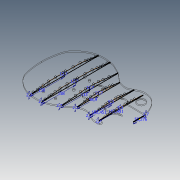
# Autodesk Inventor part: Tampo2
Saved by Autodesk Inventor 2016 (Build 200138000, 138)
## iProperties
Created: 2018-10-29
Part Number: Tampo2
Material: Generic
Document SubType Name: Modeling
Designer: Pedro Mendonça
Density: 1 g/cm^3
Appearance: Default
Author: Pedro Mendonça
Autodesk Inventor part; units mm, degrees
ref_plane "YZ Plane" through (0, 0, 0) normal (1, 0, 0) x (0, 1, 0)
ref_plane "XY Plane" through (0, 0, 0) normal (0, 0, 1) x (1, 0, 0)
sketch "Sketch1" plane through (0, 0, 0) normal (0, 0, 1) x (1, 0, 0)
  circle A0 centre (34.423, -78.21) radius 1
  circle A1 centre (41.5, -294) radius 4.5
  circle A2 centre (-41.5, -294) radius 4.5
  circle A3 centre (-36.7, -267.7941) radius 4.5
  circle A4 centre (36.7, -267.7941) radius 4.5
  line L0 (35, -127.21) -> (-13.5738, -127.21)
  line L1 (33.9001, -190.21) -> (35, -190.21)
  arc A5 (39, -194.21) -> (35, -190.21) centre (35, -194.21) ccw
  line L2 (39, -194.21) -> (39, -196.9778)
  line L3 (41.0589, -199.71) -> (41.5, -199.71)
  arc A6 (43.5, -201.71) -> (41.5, -199.71) centre (41.5, -201.71) ccw
  line L4 (43.5, -201.71) -> (43.5, -202.9495)
  arc A7 (35, -232.21) -> (38.6777, -229.783) centre (35, -228.21) ccw
  line L5 (35, -232.21) -> (-35, -232.21)
  arc A8 (-39, -228.21) -> (-35, -232.21) centre (-35, -228.21) ccw
  line L6 (-39, -228.21) -> (-39, -224.71)
  arc A9 (-39, -224.71) -> (-41, -222.71) centre (-41, -224.71) ccw
  line L7 (-41, -222.71) -> (-41.5, -222.71)
  arc A10 (-43.5, -220.71) -> (-41.5, -222.71) centre (-41.5, -220.71) ccw
  line L8 (-43.5, -220.71) -> (-43.5, -201.71)
  arc A11 (-41.5, -199.71) -> (-43.5, -201.71) centre (-41.5, -201.71) ccw
  line L9 (-41.5, -199.71) -> (-41, -199.71)
  arc A12 (-41, -199.71) -> (-39, -197.71) centre (-41, -197.71) ccw
  line L10 (-39, -197.71) -> (-39, -194.21)
  arc A13 (-35, -190.21) -> (-39, -194.21) centre (-35, -194.21) ccw
  line L11 (-35, -190.21) -> (8.8574, -190.21)
  arc A14 (-55.8091, -71.1619) -> (-75.5317, -78.2219) centre (-70.5, -61.2) ccw
  arc A15 (-39.1003, -93.3353) -> (-39, -92.71) centre (-41, -92.71) ccw
  line L12 (-39, -92.71) -> (-39, -89.21)
  arc A16 (-35, -85.21) -> (-39, -89.21) centre (-35, -89.21) ccw
  line L13 (-35, -85.21) -> (-28.53, -85.21)
  line L14 (-28.53, -85.21) -> (-27.2617, -2.2163)
  spline S0 degree 4 poles (-27.2617, -2.2163) (-43.8413, -5.0737) (-69.2989, -15.2577) (-85.7631, -26.5127) (-99.6977, -40.3072) (-106.7365, -51.5397) (-111.6352, -63.1761) (-114.1418, -74.0378) (-115.9364, -86.2479) (-114.7925, -100.8201) (-111.1925, -111.3398) (-104.9533, -123.6353) (-99.2411, -132.3298) (-94.3304, -141.7669) (-90.7434, -152.656) (-92.8358, -167.4735) (-95.3552, -177.4658) (-100.5222, -191.8137) (-106.2015, -200.3968) (-115.9364, -209.2361) (-126.4423, -222.6445) (-135, -233.5666) (-138.9752, -242.9989) (-144.1012, -253.4714) (-148.4765, -261.546) (-152.3095, -270.0787) (-155.7121, -278.8181) (-157.4845, -291.3466) (-158.9541, -299.1238) (-160.7041, -310.0555) (-161.3959, -321.0408) (-160.2622, -336.1037) (-159.5472, -351.6393) (-155.7121, -363.9428) (-152.044, -373.8933) (-146.9896, -384.4071) (-140.8913, -395.5086) (-132.7759, -406.8471) (-124.2149, -416.631) (-110.5874, -430.5207) (-101.5897, -436.4609) (-90.9559, -441.7244) (-72.5, -447.3805) (-55.0288, -449.8264) (-39.9161, -452.9713) (-21.0472, -455.5046) (0, -455) knots 1.260865 1.260865 1.260865 1.260865 1.260865 2 2.830975 3 3.639707 4 5 5.266438 6 6.852799 7 7.750355 8 8.949877 9 10 10.263862 11 11.607775 12 12.940348 13 13.693379 14 14.438323 15 15.641425 16 16.183585 17 18 19 19.17802 19.513385 20 20.856717 21 21.323358 21.522075 21.533515 21.674547 21.764236 21.807897 22 22 22 22 22
  spline S1 degree 4 poles (0, -455) (21.0472, -455.5046) (39.9161, -452.9713) (55.0288, -449.8264) (72.5, -447.3805) (90.9559, -441.7244) (101.5897, -436.4609) (110.5874, -430.5207) (124.2149, -416.631) (132.7759, -406.8471) (140.8913, -395.5086) (146.9896, -384.4071) (152.044, -373.8933) (155.7121, -363.9428) (159.5472, -351.6393) (160.2622, -336.1037) (161.3959, -321.0408) (160.7041, -310.0555) (158.9541, -299.1238) (157.4845, -291.3466) (155.7121, -278.8181) (152.3095, -270.0787) (148.4765, -261.546) (144.1012, -253.4714) (138.9752, -242.9989) (135, -233.5666) (126.4423, -222.6445) (115.9364, -209.2361) (106.2015, -200.3968) (100.5222, -191.8137) (95.3552, -177.4658) (92.8358, -167.4735) (90.7434, -152.656) (94.3304, -141.7669) (99.2411, -132.3298) (104.9533, -123.6353) (111.1925, -111.3398) (114.7925, -100.8201) (115.7876, -88.1434) (114.9001, -79.7366) (114.1554, -75.2406) (113.4907, -72.1039) knots 1 1 1 1 1 1.192103 1.235764 1.325453 1.466485 1.477925 1.676642 2 2.143283 3 3.486615 3.82198 4 5 6 6.816415 7 7.358575 8 8.561677 9 9.306621 10 10.059652 11 11.392225 12 12.736138 13 14 14.050123 15 15.249645 16 16.147201 17 17.733562 18 18.628908 18.628908 18.628908 18.628908 18.628908
  arc A17 (113.4907, -72.1039) -> (102.4514, -70.3024) centre (107.621, -73.3478) ccw
  arc A18 (28.0139, -51.4408) -> (102.4514, -70.3024) centre (67.9874, -50) ccw
  line L15 (28.0139, -51.4408) -> (28.53, -85.21)
  line L16 (28.53, -85.21) -> (35, -85.21)
  arc A19 (39, -89.21) -> (35, -85.21) centre (35, -89.21) ccw
  line L17 (39, -89.21) -> (39, -92.71)
  arc A20 (39, -92.71) -> (41, -94.71) centre (41, -92.71) ccw
  line L18 (41, -94.71) -> (41.5, -94.71)
  arc A21 (43.5, -96.71) -> (41.5, -94.71) centre (41.5, -96.71) ccw
  line L19 (43.5, -96.71) -> (43.5, -115.71)
  arc A22 (41.5, -117.71) -> (43.5, -115.71) centre (41.5, -115.71) ccw
  line L20 (41.5, -117.71) -> (41, -117.71)
  arc A23 (41, -117.71) -> (39, -119.71) centre (41, -119.71) ccw
  line L21 (39, -119.71) -> (39, -123.21)
  arc A24 (35, -127.21) -> (39, -123.21) centre (35, -123.21) ccw
  line L22 (-39, -123.21) -> (-39, -119.71)
  arc A25 (-39, -123.21) -> (-35, -127.21) centre (-35, -123.21) ccw
  line L23 (35, -127.21) -> (-35, -127.21)
  arc A26 (35, -127.21) -> (39, -123.21) centre (35, -123.21) ccw
  line L24 (39, -119.71) -> (39, -123.21)
  arc A27 (41, -117.71) -> (39, -119.71) centre (41, -119.71) ccw
  line L25 (41.5, -117.71) -> (41, -117.71)
  arc A28 (41.5, -117.71) -> (43.5, -115.71) centre (41.5, -115.71) ccw
  line L26 (43.5, -96.71) -> (43.5, -115.71)
  arc A29 (43.5, -96.71) -> (41.5, -94.71) centre (41.5, -96.71) ccw
  line L27 (41, -94.71) -> (41.5, -94.71)
  arc A30 (39, -92.71) -> (41, -94.71) centre (41, -92.71) ccw
  line L28 (39, -89.21) -> (39, -92.71)
  arc A31 (39, -89.21) -> (35, -85.21) centre (35, -89.21) ccw
  arc A32 (-35, -85.21) -> (-39, -89.21) centre (-35, -89.21) ccw
  line L29 (-39, -92.71) -> (-39, -89.21)
  arc A33 (-41, -94.71) -> (-39, -92.71) centre (-41, -92.71) ccw
  line L30 (-41.5, -94.71) -> (-41, -94.71)
  arc A34 (-41.5, -94.71) -> (-43.5, -96.71) centre (-41.5, -96.71) ccw
  line L31 (-43.5, -115.71) -> (-43.5, -96.71)
  arc A35 (-43.5, -115.71) -> (-41.5, -117.71) centre (-41.5, -115.71) ccw
  line L32 (-41, -117.71) -> (-41.5, -117.71)
  arc A36 (-39, -119.71) -> (-41, -117.71) centre (-41, -119.71) ccw
  line L33 (-39, -228.21) -> (-39, -224.71)
  arc A37 (-39, -228.21) -> (-35, -232.21) centre (-35, -228.21) ccw
  line L34 (35, -232.21) -> (-35, -232.21)
  arc A38 (35, -232.21) -> (39, -228.21) centre (35, -228.21) ccw
  line L35 (39, -224.71) -> (39, -228.21)
  arc A39 (41, -222.71) -> (39, -224.71) centre (41, -224.71) ccw
  line L36 (41.5, -222.71) -> (41, -222.71)
  arc A40 (41.5, -222.71) -> (43.5, -220.71) centre (41.5, -220.71) ccw
  line L37 (43.5, -201.71) -> (43.5, -220.71)
  arc A41 (43.5, -201.71) -> (41.5, -199.71) centre (41.5, -201.71) ccw
  line L38 (41, -199.71) -> (41.5, -199.71)
  arc A42 (39, -197.71) -> (41, -199.71) centre (41, -197.71) ccw
  line L39 (39, -194.21) -> (39, -197.71)
  arc A43 (39, -194.21) -> (35, -190.21) centre (35, -194.21) ccw
  line L40 (-35, -190.21) -> (35, -190.21)
  arc A44 (-35, -190.21) -> (-39, -194.21) centre (-35, -194.21) ccw
  line L41 (-39, -197.71) -> (-39, -194.21)
  arc A45 (-41, -199.71) -> (-39, -197.71) centre (-41, -197.71) ccw
  line L42 (-41.5, -199.71) -> (-41, -199.71)
  arc A46 (-41.5, -199.71) -> (-43.5, -201.71) centre (-41.5, -201.71) ccw
  line L43 (-43.5, -220.71) -> (-43.5, -201.71)
  arc A47 (-43.5, -220.71) -> (-41.5, -222.71) centre (-41.5, -220.71) ccw
  line L44 (-41, -222.71) -> (-41.5, -222.71)
  arc A48 (-39, -224.71) -> (-41, -222.71) centre (-41, -224.71) ccw
  arc A49 (-55.8091, -71.1619) -> (-75.5317, -78.2219) centre (-70.5, -61.2) ccw
  arc A50 (-75.5317, -78.2219) -> (-55.8091, -71.1619) centre (-70.5, -61.2) ccw
  circle A51 centre (74, -297.4128) radius 3.7
  circle A52 centre (113.9223, -275.0602) radius 3.7
  circle A53 centre (113.9223, -331.1092) radius 3.7
  circle A54 centre (74, -348.8838) radius 3.7
  line L45 (-35, -85.21) -> (-28.53, -85.21)
  line L46 (28.53, -85.21) -> (35, -85.21)
  point P0 (0, 0)
  point P1 (0, 0)
  constraints: 94 end point, 92 point on circle, 55 centre point, 4 other
extrude "base" add sketch "Sketch1" along normal blind 5.4
ref_plane "Work Plane1" through (-28.53, -85.21, 5.4) normal (0, 1, 0) x (-1, 0, 0)
ref_plane "Work Plane2" through (0, -127.21, 5.4) normal (0, 1, 0) x (-1, 0, 0)
ref_plane "Work Plane3" through (0, -190.21, 0) normal (0, 1, 0) x (-1, 0, 0)
ref_plane "Work Plane4" through (0, -232.21, 0) normal (0, 1, 0) x (-1, 0, 0)
ref_plane "Work Plane5" through (41.5, -294, 5.4) normal (0, 1, 0) x (-1, 0, 0)
ref_plane "Work Plane6" through (74, -348.8838, 0) normal (0, 1, 0) x (-1, 0, 0)
sketch "Sketch2" plane through (0, 0, 0) normal (0, 1, 0) x (-1, 0, 0)
  line L0 (-28.0139, 5.4) -> (27.2617, 5.4)
  line L1 (27.2617, 5.4) -> (27.2617, 2.7)
  line L2 (-28.0139, 5.4) -> (-28.0139, 2.7)
  line L3 (-28.0139, 2.7) -> (27.2617, 2.7)
  point P0 (0, 0)
  dimension "d45" = 2.7
  dimension "d46" = 55.2756
  constraints: 8 end point, 2 horizontal, 1 perpendicular, 1 point on line
  measures "d45" distance of L0.end L1.end
  measures "d46" distance of L2.end L1.end
sketch "Sketch3" plane through (-28.53, -85.21, 5.4) normal (0, 1, 0) x (-1, 0, 0)
  line L0 (-28.53, -2.7) -> (-28.53, 2.6)
  line L1 (-28.53, -2.7) -> (-28.53, 0)
  line L2 (-28.53, 0) -> (-131.03, 0) construction
  line L3 (-130.9814, -2.7) -> (-130.9814, 0)
  line L4 (-130.9814, 0) -> (-90.7981, 1.127) construction
  line L5 (-90.7981, 1.127) -> (-77.2588, 1.5284) construction
  line L6 (-77.2588, 1.5284) -> (-60.9572, 1.5284) construction
  line L7 (-60.9572, 1.5284) -> (-46.9035, 2.6) construction
  line L8 (-46.9035, 2.6) -> (-28.53, 2.6) construction
  spline S0 degree 4 poles (-130.9814, 0) (-90.7981, 1.127) (-77.2588, 1.5284) (-60.9572, 1.5284) (-46.9035, 2.6) (-28.53, 2.6) knots 1 1 1 1 1 2 3 3 3 3 3
  line L9 (-130.9814, 0) -> (-130.9814, -2.7)
  line L10 (-130.9814, 0) -> (-125.5814, 0) construction
  line L11 (-130.9814, -2.7) -> (-28.53, -2.7)
  line L12 (-28.53, 0) -> (73.97, 0) construction
  line L13 (73.9214, -2.7) -> (73.9214, 0)
  line L14 (73.9214, 0) -> (33.7381, 1.127) construction
  spline S1 degree 4 poles (73.9214, 0) (33.7381, 1.127) (20.1988, 1.5284) (3.8972, 1.5284) (-10.1565, 2.6) (-28.53, 2.6) knots 1 1 1 1 1 2 3 3 3 3 3
  line L15 (33.7381, 1.127) -> (20.1988, 1.5284) construction
  line L16 (20.1988, 1.5284) -> (3.8972, 1.5284) construction
  line L17 (3.8972, 1.5284) -> (-10.1565, 2.6) construction
  line L18 (-10.1565, 2.6) -> (-28.53, 2.6) construction
  line L19 (73.9214, 0) -> (73.9214, -2.7)
  line L20 (73.9214, 0) -> (68.5214, 0) construction
  line L21 (73.9214, -2.7) -> (-28.53, -2.7)
  point P0 (-28.53, -5.4)
  dimension "d42" = 5.3
  dimension "d43" = 102.4514
  dimension "d44" = 2.7
  constraints: 24 end point, 8 symmetric about line, 3 horizontal, 1 collinear, 1 vertical, 6 other
  measures "d42" distance of L0.start L0.end
  measures "d43" distance of L3.start L0.start
  measures "d44" distance of L3.end L3.start
sketch "Sketch5" plane through (0, -127.21, 5.4) normal (0, 1, 0) x (-1, 0, 0)
  line L0 (0, -2.7) -> (0, 6.6)
  line L1 (0, 0) -> (-102.5, 0) construction
  line L2 (-102.4514, 0) -> (-60.1171, 1.5284) construction
  line L3 (-60.1171, 1.5284) -> (-42.8591, 3.5935) construction
  line L4 (-42.8591, 3.5935) -> (-28.8463, 5.806) construction
  line L5 (-28.8463, 5.806) -> (-18.3735, 6.6) construction
  line L6 (-18.3735, 6.6) -> (0, 6.6) construction
  spline S0 degree 4 poles (-102.4514, 0) (-60.1171, 1.5284) (-42.8591, 3.5935) (-28.8463, 5.806) (-18.3735, 6.6) (0, 6.6) knots 1 1 1 1 1 2 3 3 3 3 3
  line L7 (-102.4514, 0) -> (-102.4514, -2.7)
  line L8 (-102.4514, 0) -> (-97.0514, 0) construction
  line L9 (-102.4514, -2.7) -> (0, -2.7)
  line L10 (0, 0) -> (102.5, 0) construction
  line L11 (102.4514, 0) -> (60.1171, 1.5284) construction
  line L12 (60.1171, 1.5284) -> (42.8591, 3.5935) construction
  line L13 (42.8591, 3.5935) -> (28.8463, 5.806) construction
  line L14 (28.8463, 5.806) -> (18.3735, 6.6) construction
  line L15 (18.3735, 6.6) -> (0, 6.6) construction
  spline S1 degree 4 poles (102.4514, 0) (60.1171, 1.5284) (42.8591, 3.5935) (28.8463, 5.806) (18.3735, 6.6) (0, 6.6) knots 1 1 1 1 1 2 3 3 3 3 3
  line L16 (102.4514, 0) -> (102.4514, -2.7)
  line L17 (102.4514, 0) -> (97.0514, 0) construction
  line L18 (102.4514, -2.7) -> (0, -2.7)
  dimension "d39" = 102.4514
  dimension "d40" = 9.3
  dimension "d41" = 2.7
  constraints: 18 end point, 8 symmetric about line, 3 horizontal, 1 vertical, 6 other
  measures "d39" distance of L7.end L0.start
  measures "d40" distance of L0.start L0.end
  measures "d41" distance of L2.start L7.end
sketch "Sketch6" plane through (0, -190.21, 0) normal (0, 1, 0) x (-1, 0, 0)
  line L0 (0, 2.7) -> (0, 15.4)
  line L1 (0, 2.7) -> (0, 5.4)
  line L2 (0, 5.4) -> (-98.9, 5.4) construction
  line L3 (-98.9, 2.7) -> (-98.9, 5.4)
  line L4 (-98.9, 5.4) -> (-65.1223, 8.4413) construction
  line L5 (-65.1223, 8.4413) -> (-51.5336, 11.3544) construction
  line L6 (-51.5336, 11.3544) -> (-35.6571, 12.4274) construction
  line L7 (-35.6571, 12.4274) -> (-18.3735, 15.4) construction
  line L8 (-18.3735, 15.4) -> (0, 15.4) construction
  spline S0 degree 4 poles (-98.9, 5.4) (-65.1223, 8.4413) (-51.5336, 11.3544) (-35.6571, 12.4274) (-18.3735, 15.4) (0, 15.4) knots 1 1 1 1 1 2 3 3 3 3 3
  line L9 (-102.4514, 5.4) -> (-97.0514, 5.4) construction
  line L10 (-98.9, 2.7) -> (0, 2.7)
  line L11 (0, 5.4) -> (98.9, 5.4) construction
  line L12 (98.9, 2.7) -> (98.9, 5.4)
  line L13 (98.9, 5.4) -> (65.1223, 8.4413) construction
  spline S1 degree 4 poles (98.9, 5.4) (65.1223, 8.4413) (51.5336, 11.3544) (35.6571, 12.4274) (18.3735, 15.4) (0, 15.4) knots 1 1 1 1 1 2 3 3 3 3 3
  line L14 (65.1223, 8.4413) -> (51.5336, 11.3544) construction
  line L15 (51.5336, 11.3544) -> (35.6571, 12.4274) construction
  line L16 (35.6571, 12.4274) -> (18.3735, 15.4) construction
  line L17 (18.3735, 15.4) -> (0, 15.4) construction
  line L18 (102.4514, 5.4) -> (97.0514, 5.4) construction
  line L19 (98.9, 2.7) -> (0, 2.7)
  point P0 (0, 0)
  dimension "d36" = 12.7
  dimension "d37" = 98.9
  dimension "d38" = 2.7
  constraints: 20 end point, 9 symmetric about line, 3 horizontal, 1 collinear, 6 other
  measures "d36" distance of L0.start L0.end
  measures "d37" distance of L3.start L0.start
  measures "d38" distance of L3.start L3.end
sketch "Sketch7" plane through (0, -232.21, 0) normal (0, 1, 0) x (-1, 0, 0)
  line L0 (0, 2.7) -> (0, 15.4)
  line L1 (0, 0) -> (0, 5.4)
  line L2 (-133, 5.4) -> (-91.8421, 7.7) construction
  spline S0 degree 4 poles (-133, 5.4) (-91.8421, 7.7) (-64.2725, 11.1458) (-41.6932, 13.9678) (-18.3735, 15.4) (0, 15.4) knots 1 1 1 1 1 2 3 3 3 3 3
  line L3 (-91.8421, 7.7) -> (-64.2725, 11.1458) construction
  line L4 (-64.2725, 11.1458) -> (-41.6932, 13.9678) construction
  line L5 (-41.6932, 13.9678) -> (-18.3735, 15.4) construction
  line L6 (-18.3735, 15.4) -> (0, 15.4) construction
  line L7 (-102.4514, 5.4) -> (-97.0514, 5.4) construction
  line L8 (-133, 2.7) -> (-133, 5.4)
  line L9 (-133, 2.7) -> (0, 2.7)
  line L10 (133, 5.4) -> (91.8421, 7.7) construction
  spline S1 degree 4 poles (133, 5.4) (91.8421, 7.7) (64.2725, 11.1458) (41.6932, 13.9678) (18.3735, 15.4) (0, 15.4) knots 1 1 1 1 1 2 3 3 3 3 3
  line L11 (91.8421, 7.7) -> (64.2725, 11.1458) construction
  line L12 (64.2725, 11.1458) -> (41.6932, 13.9678) construction
  line L13 (41.6932, 13.9678) -> (18.3735, 15.4) construction
  line L14 (18.3735, 15.4) -> (0, 15.4) construction
  line L15 (102.4514, 5.4) -> (97.0514, 5.4) construction
  line L16 (133, 2.7) -> (133, 5.4)
  line L17 (133, 2.7) -> (0, 2.7)
  point P0 (0, 0)
  dimension "d33" = 133
  dimension "d34" = 12.7
  dimension "d35" = 2.7
  constraints: 16 end point, 8 symmetric about line, 3 horizontal, 1 collinear, 1 midpoint, 1 vertical, 6 other
  measures "d33" distance of L8.start L0.start
  measures "d34" distance of L0.start L0.end
  measures "d35" distance of L8.start L2.start
sketch "Sketch8" plane through (41.5, -294, 5.4) normal (0, 1, 0) x (-1, 0, 0)
  line L0 (41.5, -2.7) -> (41.5, 10)
  line L1 (41.5, -2.7) -> (41.5, 0)
  line L2 (-116.5, 0) -> (-103.2049, 0.4658) construction
  spline S0 degree 4 poles (-116.5, 0) (-103.2049, 0.4658) (-83.9092, 1.9932) (-71.0129, 2.6649) (-55.5514, 5.9842) (-32.4504, 9.4738) (0.236, 10) (35.8809, 10) (41.5, 10) knots 1 1 1 1 1 2 2.205504 2.599053 2.694176 3 3 3 3 3
  line L3 (-103.2049, 0.4658) -> (-83.9092, 1.9932) construction
  line L4 (35.8809, 10) -> (41.5, 10) construction
  line L5 (-60.9514, 0) -> (-55.5514, 0) construction
  line L6 (-116.5, -2.7) -> (-116.5, 0)
  line L7 (-83.9092, 1.9932) -> (-71.0129, 2.6649) construction
  line L8 (-71.0129, 2.6649) -> (-55.5514, 5.9842) construction
  line L9 (-55.5514, 5.9842) -> (-32.4504, 9.4738) construction
  line L10 (-32.4504, 9.4738) -> (0.236, 10) construction
  line L11 (0.236, 10) -> (35.8809, 10) construction
  line L12 (-116.5, -2.7) -> (41.5, -2.7)
  line L13 (199.5, 0) -> (186.2049, 0.4658) construction
  spline S1 degree 4 poles (199.5, 0) (186.2049, 0.4658) (166.9092, 1.9932) (154.0129, 2.6649) (138.5514, 5.9842) (115.4504, 9.4738) (82.764, 10) (47.1191, 10) (41.5, 10) knots 1 1 1 1 1 2 2.205504 2.599053 2.694176 3 3 3 3 3
  line L14 (186.2049, 0.4658) -> (166.9092, 1.9932) construction
  line L15 (47.1191, 10) -> (41.5, 10) construction
  line L16 (143.9514, 0) -> (138.5514, 0) construction
  line L17 (199.5, -2.7) -> (199.5, 0)
  line L18 (166.9092, 1.9932) -> (154.0129, 2.6649) construction
  line L19 (154.0129, 2.6649) -> (138.5514, 5.9842) construction
  line L20 (138.5514, 5.9842) -> (115.4504, 9.4738) construction
  line L21 (115.4504, 9.4738) -> (82.764, 10) construction
  line L22 (82.764, 10) -> (47.1191, 10) construction
  line L23 (199.5, -2.7) -> (41.5, -2.7)
  point P0 (41.5, -5.4)
  point P1 (41.5, -5.4)
  point P2 (41.5, -5.4)
  point P3 (-116.5, -5.4)
  point P4 (199.5, -5.4)
  dimension "d30" = 158
  dimension "d31" = 12.7
  dimension "d32" = 2.7
  constraints: 16 end point, 12 symmetric about line, 3 horizontal, 1 collinear, 1 vertical, 6 other
  measures "d30" distance of L6.start L0.start
  measures "d31" distance of L0.start L0.end
  measures "d32" distance of L6.start L2.start
sketch "Sketch9" plane through (74, -348.8838, 0) normal (0, 1, 0) x (-1, 0, 0)
  line L0 (74, 2.7) -> (74, 15.4)
  line L1 (74, 2.7) -> (74, 5.4)
  line L2 (-84, 5.4) -> (-70.7049, 5.8658) construction
  spline S0 degree 4 poles (-84, 5.4) (-70.7049, 5.8658) (-51.4092, 7.3932) (-38.5129, 8.0649) (-24.9094, 12.2215) (0.0496, 14.8738) (32.736, 15.4) (68.3809, 15.4) (74, 15.4) knots 1 1 1 1 1 2 2.205504 2.599053 2.694176 3 3 3 3 3
  line L3 (-70.7049, 5.8658) -> (-51.4092, 7.3932) construction
  line L4 (68.3809, 15.4) -> (74, 15.4) construction
  line L5 (-28.4514, 5.4) -> (-23.0514, 5.4) construction
  line L6 (-84, 2.7) -> (-84, 5.4)
  line L7 (-51.4092, 7.3932) -> (-38.5129, 8.0649) construction
  line L8 (-38.5129, 8.0649) -> (-24.9094, 12.2215) construction
  line L9 (-24.9094, 12.2215) -> (0.0496, 14.8738) construction
  line L10 (0.0496, 14.8738) -> (32.736, 15.4) construction
  line L11 (32.736, 15.4) -> (68.3809, 15.4) construction
  line L12 (199.4092, 7.3932) -> (186.5129, 8.0649) construction
  spline S1 degree 4 poles (232, 5.4) (218.7049, 5.8658) (199.4092, 7.3932) (186.5129, 8.0649) (172.9094, 12.2215) (147.9504, 14.8738) (115.264, 15.4) (79.6191, 15.4) (74, 15.4) knots 1 1 1 1 1 2 2.205504 2.599053 2.694176 3 3 3 3 3
  line L13 (232, 5.4) -> (218.7049, 5.8658) construction
  line L14 (218.7049, 5.8658) -> (199.4092, 7.3932) construction
  line L15 (186.5129, 8.0649) -> (172.9094, 12.2215) construction
  line L16 (172.9094, 12.2215) -> (147.9504, 14.8738) construction
  line L17 (147.9504, 14.8738) -> (115.264, 15.4) construction
  line L18 (115.264, 15.4) -> (79.6191, 15.4) construction
  line L19 (79.6191, 15.4) -> (74, 15.4) construction
  line L20 (232, 0) -> (232, 5.4)
  line L21 (176.4514, 5.4) -> (171.0514, 5.4) construction
  line L22 (74, 2.7) -> (-84, 2.7)
  line L23 (232, 5.4) -> (218.7049, 5.8658) construction
  spline S2 degree 4 poles (232, 5.4) (218.7049, 5.8658) (199.4092, 7.3932) (186.5129, 8.0649) (172.9094, 12.2215) (147.9504, 14.8738) (115.264, 15.4) (79.6191, 15.4) (74, 15.4) knots 1 1 1 1 1 2 2.205504 2.599053 2.694176 3 3 3 3 3
  line L24 (218.7049, 5.8658) -> (199.4092, 7.3932) construction
  line L25 (199.4092, 7.3932) -> (186.5129, 8.0649) construction
  line L26 (186.5129, 8.0649) -> (172.9094, 12.2215) construction
  line L27 (172.9094, 12.2215) -> (147.9504, 14.8738) construction
  line L28 (147.9504, 14.8738) -> (115.264, 15.4) construction
  line L29 (115.264, 15.4) -> (79.6191, 15.4) construction
  line L30 (79.6191, 15.4) -> (74, 15.4) construction
  line L31 (176.4514, 5.4) -> (171.0514, 5.4) construction
  line L32 (232, 2.7) -> (232, 5.4)
  line L33 (74, 2.7) -> (232, 2.7)
  point P0 (74, 2.7)
  point P1 (74, 0)
  point P2 (74, 0)
  point P3 (-84, 0)
  dimension "d27" = 12.7
  dimension "d28" = 2.7
  dimension "d29" = 158
  constraints: 20 end point, 12 symmetric about line, 3 horizontal, 1 coincident, 1 collinear, 1 vertical, 9 other
  measures "d27" distance of L0.start L0.end
  measures "d28" distance of L6.start L2.start
  measures "d29" distance of L0.start L6.start
body "Solid1"
